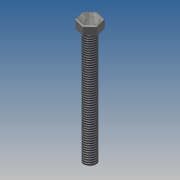
# Autodesk Inventor part: lagBolt_38
Saved by Autodesk Inventor 2014 SP1 (Build 180222100, 222)
## iProperties
Created: 2014-08-29
Part Number: lagBolt_38
Material: Steel, Galvanized
Document SubType Name: Modeling
Designer: Dave
Density: 7.85 g/cm^3
Appearance: Galvanized
Mass: 40.1345 g
Surface Area: 23.6147 cm^2
Volume: 5.11267 cm^3
Author: Dave
Autodesk Inventor part; units mm, degrees
ref_plane "YZ Plane" through (0, 0, 0) normal (1, 0, 0) x (0, 1, 0)
ref_plane "XZ Plane" through (0, 0, 0) normal (0, 1, 0) x (-1, 0, 0)
ref_plane "XY Plane" through (0, 0, 0) normal (0, 0, 1) x (1, 0, 0)
sketch "Sketch1" plane through (0, 0, 0) normal (0, 1, 0) x (-1, 0, 0)
  line L0 (-2.027, 7.8067) -> (5.7473, 5.6588)
  line L1 (5.7473, 5.6588) -> (7.7743, -2.1479)
  line L2 (7.7743, -2.1479) -> (2.027, -7.8067)
  line L3 (2.027, -7.8067) -> (-5.7473, -5.6588)
  line L4 (-5.7473, -5.6588) -> (-7.7743, 2.1479)
  line L5 (-7.7743, 2.1479) -> (-2.027, 7.8067)
  point P0 (0, 0)
  point P1 (0, 0)
  dimension "d8" = 13.97
  constraints: 12 end point, 1 coincident, 13 other
  measures "d8" distance between parallel lines of L1 L4
extrude "Extrusion1" add sketch "Sketch1" along normal blind 6.35
fillet "Fillet1" radius 0.762 6 edges at (4.9007, 6.35, 4.9773) (6.7608, 6.35, -1.7554) (1.8602, 6.35, -6.7328) (-4.9007, 6.35, -4.9773) (-6.7608, 6.35, 1.7554) (-1.8602, 6.35, 6.7328)
sketch "Sketch2" plane through (0, 0, 0) normal (0, -1, 0) x (1, 0, 0)
  circle A0 centre (0, 0) radius 4.6482
  dimension "d3" = 9.2964
  constraints: 1 centre point, 1 coincident
  measures "d3" diameter of A0
extrude "Extrusion2" add sketch "Sketch2" along normal blind 88.9
thread "Thread1" size "3/8-16 UNC" class "2A" standard "ANSI Unified Screw Threads" full length
body "Solid1"
